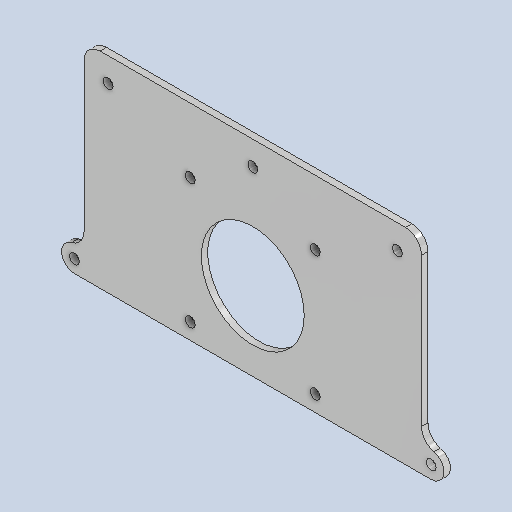
# Autodesk Inventor part: omu_al_jo_1
Saved by Autodesk Inventor 2025.2 (Build 292293000, 293)
## iProperties
Created: 2024-03-23
Part Number: omu_al_jo_1
Material: アルミニウム 6061-AHC
Document SubType Name: Modeling
Designer: fhbdh
Density: 2.7 g/cm^3
Appearance: アルミニウム - ダーク
Author: fhbdh
Autodesk Inventor part; units mm, degrees
ref_plane "YZ Plane" through (0, 0, 0) normal (1, 0, 0) x (0, 1, 0)
ref_plane "XZ Plane" through (0, 0, 0) normal (0, 1, 0) x (-1, 0, 0)
ref_plane "XY Plane" through (0, 0, 0) normal (0, 0, 1) x (1, 0, 0)
sketch "スケッチ1" plane through (0, 0, 0) normal (0, 0, 1) x (1, 0, 0)
  circle A0 centre (0, 0) radius 52.5 construction
  circle A1 centre (0, 0) radius 12.55 construction
  circle A2 centre (-12.3744, 12.3744) radius 2.05 construction
  circle A3 centre (-12.3744, -12.3744) radius 2.05 construction
  circle A4 centre (12.3744, -12.3744) radius 2.05 construction
  circle A5 centre (12.3744, 12.3744) radius 2.05 construction
  line L0 (0, 0) -> (-12.3744, 12.3744) construction
  line L1 (0, 0) -> (0, 12.55) construction
  circle A6 centre (0, 0) radius 23.5 construction
  line L2 (-52.5, 39.5) -> (52.5, 39.5)
  line L3 (52.5, 39.5) -> (52.5, -24.4454)
  line L4 (52.5, -24.4454) -> (-52.5, -24.4454)
  line L5 (-52.5, -24.4454) -> (-52.5, 39.5)
  line L6 (-52.5, 24.5) -> (52.5, 24.5) construction
  line L7 (-52.5, 32) -> (52.5, 32) construction
  circle A7 centre (0, 32) radius 1.55
  circle A8 centre (-45, 32) radius 1.55
  circle A9 centre (45, 32) radius 1.55
  circle A10 centre (-19.4454, 19.4454) radius 1.55
  circle A11 centre (-19.4454, -19.4454) radius 1.55
  circle A12 centre (19.4454, -19.4454) radius 1.55
  circle A13 centre (19.4454, 19.4454) radius 1.55
  line L8 (-52.5, -24.4454) -> (-55.5, -24.4454)
  circle A14 centre (-55.5, -20.4454) radius 1.55
  arc A15 (-55.5, -16.4454) -> (-55.5, -24.4454) centre (-55.5, -20.4454) ccw
  line L9 (-55.5, -16.4454) -> (-52.5, -16.4454)
  line L10 (52.5, -24.4454) -> (55.5, -24.4454)
  circle A16 centre (55.5, -20.4454) radius 1.55
  arc A17 (55.5, -24.4454) -> (55.5, -16.4454) centre (55.5, -20.4454) ccw
  line L11 (55.5, -16.4454) -> (52.5, -16.4454)
  circle A18 centre (0, 0) radius 16
  point P0 (0, 39.5)
  point P1 (0, 23.5)
  point P2 (0, -52.5)
  dimension "d0" = 105
  dimension "d1" = 25.1
  dimension "d9" = 47
  dimension "d2" = 4.1
  dimension "d5" = 360
  dimension "d7" = 45
  dimension "d8" = 35
  dimension "d10" = 15
  dimension "d18" = 105
  dimension "d20" = 7.5
  dimension "d21" = 3.1
  dimension "d22" = 3.1
  dimension "d23" = 3.1
  dimension "d24" = 90
  dimension "d27" = 3.1
  dimension "d30" = 360
  dimension "d32" = 55
  dimension "d33" = 5
  dimension "d35" = 3.1
  dimension "d36" = 4
  dimension "d37" = 3
  dimension "d38" = 32
  dimension "d40" = 92
  constraints: 24 end point, 16 centre point, 12 point on line, 6 coincident, 6 symmetric about line, 4 perpendicular, 4 point on circle, 3 vertical alignment, 2 horizontal, 2 midpoint, 2 parallel, 2 tangent, 1 vertical, 26 other
  measures "d2" diameter of A2
  measures "d7" angle of L1 L0
  measures "d8" distance of A4.centre L0.end
  measures "d10" distance between parallel lines of L6 L2
  measures "d18" distance of L2.start L2.end
  measures "d20" distance between parallel lines of L2 L7
  measures "d21" diameter of A7
  measures "d22" diameter of A8
  measures "d23" diameter of A9
  measures "d24" distance of A9.centre A8.centre
  measures "d27" diameter of A10
  measures "d32" distance of A12.centre A10.centre
  measures "d33" distance from line of L4 A11.centre
  measures "d35" diameter of A14
  measures "d36" radius of A15
  measures "d37" distance of L9.start L9.end
  measures "d38" diameter of A18
  measures "d40" distance from line of point (0, -52.5) L2
extrude "押し出し1" add sketch "スケッチ1" along normal blind 2
fillet "フィレット1" radius 5 4 edges at (-52.5, 39.5, 1) (52.5, 39.5, 1) (52.5, -16.4454, 1) (-52.5, -16.4454, 1)
sketch "スケッチ2" plane through (0, 0, 2) normal (0, 0, 1) x (1, 0, 0)
  arc A0 (52.5, 34.5) -> (47.5, 39.5) centre (47.5, 34.5) ccw projected
  line L0 (47.5, 39.5) -> (-47.5, 39.5) projected
  arc A1 (-47.5, 39.5) -> (-52.5, 34.5) centre (-47.5, 34.5) ccw projected
  line L1 (-52.5, 34.5) -> (-52.5, -11.6705) projected
  arc A2 (-56.3889, -16.5455) -> (-52.5, -11.6705) centre (-57.5, -11.6705) ccw projected
  arc A3 (-56.3889, -16.5455) -> (-55.5, -24.4454) centre (-55.5, -20.4454) ccw projected
  line L2 (-55.5, -24.4454) -> (55.5, -24.4454) projected
  arc A4 (55.5, -24.4454) -> (56.3889, -16.5455) centre (55.5, -20.4454) ccw projected
  arc A5 (52.5, -11.6705) -> (56.3889, -16.5455) centre (57.5, -11.6705) ccw projected
  line L3 (52.5, -11.6705) -> (52.5, 34.5) projected
  circle A6 centre (-55.5, -20.4454) radius 1.55 projected
  circle A7 centre (0, 0) radius 16 projected
  circle A8 centre (19.4454, -19.4454) radius 1.55 projected
  circle A9 centre (-19.4454, -19.4454) radius 1.55 projected
  circle A10 centre (-19.4454, 19.4454) radius 1.55 projected
  circle A11 centre (45, 32) radius 1.55 projected
  circle A12 centre (-45, 32) radius 1.55 projected
  circle A13 centre (0, 32) radius 1.55 projected
  circle A14 centre (19.4454, 19.4454) radius 1.55 projected
  circle A15 centre (55.5, -20.4454) radius 1.55 projected
equation "\"d20\" = 0.5 * d10"
